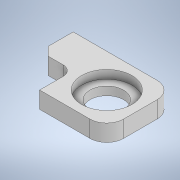
# Autodesk Inventor part: Peça4
Saved by Autodesk Inventor 2021 (Build 250183000, 183)
## iProperties
Created: 2022-02-15
Part Number: Peça4
Material: Genérico
Document SubType Name: Modeling
Designer: aluno
Density: 1 g/cm^3
Appearance: Padrão
Author: aluno
Autodesk Inventor part; units mm, degrees
ref_plane "YZ Plane" through (0, 0, 0) normal (1, 0, 0) x (0, 1, 0)
ref_plane "XZ Plane" through (0, 0, 0) normal (0, 1, 0) x (-1, 0, 0)
ref_plane "XY Plane" through (0, 0, 0) normal (0, 0, 1) x (1, 0, 0)
sketch "Esboço1" plane through (0, 0, 0) normal (0, 1, 0) x (-1, 0, 0)
  line L0 (0, 0) -> (200, 0)
  line L1 (200, 0) -> (200, -100)
  line L2 (200, -100) -> (300, -100)
  line L3 (300, -100) -> (300, -200)
  line L4 (300, -200) -> (0, -200)
  line L5 (0, -200) -> (0, 0)
  dimension "d0" = 200
  dimension "d1" = 300
  dimension "d3" = 200
  dimension "d4" = 100
  constraints: 12 end point, 5 perpendicular, 1 horizontal
  measures "d0" distance of L0.start L0.end
  measures "d1" distance of L3.end L4.end
  measures "d3" distance of L4.end L0.start
  measures "d4" distance of L2.end L3.end
extrude "Extrusão1" add sketch "Esboço1" along normal blind 50
sketch "Esboço2" plane through (0, 50, 0) normal (0, 1, 0) x (1, 0, 0)
  line L0 (0, 0) -> (0, 200) projected
  line L1 (0, 200) -> (-300, 200) projected
  point P0 (-100, 100)
  dimension "d7" = 100
  dimension "d15" = 100
  measures "d7" distance from line of L0 point (-100, 100)
  measures "d15" distance from line of L1 point (-100, 100)
hole "Furo1" at (-100, 50, -100) direction (0, -1, 0) diameter 100 end through all counterbore diameter 150 counterbore depth 25
fillet "Arredondamento1" radius 50 2 edges at (0, 25, 0) (0, 25, -200)
fillet "Arredondamento2" radius 30 1 edges at (-200, 25, -100)
chamfer "Chanfro1" distance 25 angle 45 1 edges at (-300, 25, -100) measured on face at (-276.6667, 16.6667, -100)
equation "\"d7\" = 0.5 * d3"
equation "\"d15\" = 0.5 * d0"
equation "\"d16\" = 0.25 * d3"
